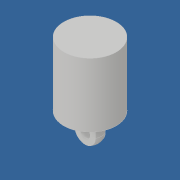
# Autodesk Inventor part: Kolben
Saved by Autodesk Inventor 2018 (Build 220112000, 112)
## iProperties
Created: 2018-09-25
Part Number: Kolben
Material: Generisch
Document SubType Name: Modeling
Designer: M.Knabel
Density: 1 g/cm^3
Appearance: Vorgabe
Author: M.Knabel
Autodesk Inventor part; units mm, degrees
ref_plane "YZ Plane" through (0, 0, 0) normal (1, 0, 0) x (0, 1, 0)
ref_plane "XZ Plane" through (0, 0, 0) normal (0, 1, 0) x (-1, 0, 0)
ref_plane "XY Plane" through (0, 0, 0) normal (0, 0, 1) x (1, 0, 0)
sketch "Skizze1" plane through (0, 0, 0) normal (0, 0, 1) x (1, 0, 0)
  line L0 (-11.2, 0) -> (11.2, 0) projected
  line L1 (0, -11.2) -> (0, 11.2) projected
  circle A0 centre (0, 0) radius 8
  dimension "d0" = 16
  constraints: 1 centre point, 1 coincident
  measures "d0" diameter of A0
extrude "Extrusion1" add sketch "Skizze1" along normal blind 19.5
sketch "Skizze2" plane through (0, 0, 0) normal (0, 1, 0) x (-1, 0, 0)
  line L0 (11.2, 0) -> (-11.2, 0) projected
  line L1 (0, -3.9) -> (0, 23.4) projected
  arc A0 (-3.5, -5) -> (3.5, -5) centre (0, -5) ccw
  line L2 (3.5, -5) -> (3.5, 0)
  line L3 (-8, 0) -> (8, 0) projected
  line L4 (-3.5, -5) -> (-3.5, 0)
  point P0 (0, 0)
  dimension "d3" = 3.5
  dimension "d4" = 5
  constraints: 4 end point, 3 point on line, 2 point on circle, 1 centre point, 1 parallel, 1 perpendicular, 1 tangent, 1 other
  measures "d3" radius of A0
  measures "d4" distance from line of L0 A0.centre
extrude "Extrusion2" add sketch "Skizze2" along normal mid plane 3
sketch "Skizze3" plane through (0, 1.5, 0) normal (0, 1, 0) x (1, 0, 0)
  arc A0 (3.5, 5) -> (-3.5, 5) centre (0, 5) ccw projected
  point P0 (0, 0)
  constraints: 1 coincident
hole "Bohrung1" at (0, 1.5, -5) direction (0, -1, 0) diameter 3 end through all
sketch "Skizze4" plane through (0, 0, 0) normal (0, 0, -1) x (-1, 0, 0)
  line L0 (-3.5, -1.5) -> (-3.5, 1.5) projected
  line L1 (3.5, -1.5) -> (3.5, 1.5) projected
  line L2 (-3.5, 1.5) -> (3.5, 1.5) projected
  line L3 (-3.5, -1.5) -> (-3.5, 1.5) projected
  line L4 (3.5, -1.5) -> (-3.5, -1.5) projected
  arc A0 (-3.1623, 1.5) -> (-3.1623, -1.5) centre (0, 0) ccw
  line L5 (-3.1623, 1.5) -> (-3.8633, 1.5)
  line L6 (-3.8633, 1.5) -> (-3.8633, -1.5)
  line L7 (-3.8633, -1.5) -> (-3.1623, -1.5)
  dimension "d14" = 3.5
  dimension "d15" = 3.8632
  constraints: 6 end point, 3 point on line, 2 point on circle, 1 centre point, 1 coincident, 1 collinear, 1 perpendicular
  measures "d14" radius of A0
  measures "d15" distance from line of L6 A0.centre
sketch "Skizze5" plane through (0, -1.5, 0) normal (0, -1, 0) x (1, 0, 0)
  arc A0 (-3.5, -5) -> (3.5, -5) centre (0, -5) ccw projected
  arc A1 (-3.5, -5) -> (3.5, -5) centre (0, -5) ccw
  line L0 (-3.5, 0) -> (-3.5, -5)
  line L1 (3.5, -5) -> (3.5, 0.5133)
  point P0 (0, 0)
  constraints: 4 end point, 2 point on circle, 2 tangent, 2 vertical, 1 centre point, 1 coincident
sketch3d "3D-Skizze1"
  line L0 (3.5, -1.5, 0) -> (3.5, -1.5, -5)
  arc A0 (-3.5, -1.5, -5) -> (-2.4749, -1.5, -7.4749) centre (0, -1.5, -5) ccw
  arc A1 (-2.4749, -1.5, -7.4749) -> (0, -1.5, -8.5) centre (0, -1.5, -5) ccw
  arc A2 (0, -1.5, -8.5) -> (2.4749, -1.5, -7.4749) centre (0, -1.5, -5) ccw
  arc A3 (2.4749, -1.5, -7.4749) -> (3.5, -1.5, -5) centre (0, -1.5, -5) ccw
  line L1 (-3.5, -1.5, -5) -> (-3.5, -1.5, 0)
sweep "Sweeping1" cut profiles "Skizze4" path "3D-Skizze1" contours L7 L6 L5 L0 | L0 A0 L4 | L0 L2 A0
